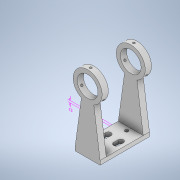
# Autodesk Inventor part: finderMainPartV05
Saved by Autodesk Inventor 2021 (Build 250183000, 183)
## iProperties
Created: 2020-06-05
Part Number: finderMainPartV05
Material: Generic
Document SubType Name: Modeling
Designer: robst
Density: 1 g/cm^3
Appearance: Default
Author: robst
Autodesk Inventor part; units mm, degrees
ref_plane "YZ Plane" through (0, 0, 0) normal (1, 0, 0) x (0, 1, 0)
ref_plane "XY Plane" through (0, 0, 0) normal (0, 0, 1) x (1, 0, 0)
sketch "Sketch1" plane through (0, 0, 0) normal (0, 0, 1) x (1, 0, 0)
  arc A0 (19.05, 73.7803) -> (-19.05, 73.7803) centre (0, 0) ccw
  line L0 (0, 86.4803) -> (19.05, 86.4803)
  line L1 (19.05, 86.4803) -> (19.05, 73.7803)
  line L2 (0, 76.2) -> (0, 86.4803) construction
  line L3 (0, 86.4803) -> (-19.05, 86.4803)
  line L4 (-19.05, 86.4803) -> (-19.05, 73.7803)
  dimension "d0" = 152.4
  dimension "d1" = 19.05
  dimension "d2" = 12.7
  constraints: 10 end point, 3 point on circle, 2 symmetric about line, 1 centre point, 1 coincident, 1 horizontal, 1 perpendicular, 1 vertical
  measures "d0" diameter of A0
  measures "d1" distance of L0.start L0.end
  measures "d2" distance of L0.end L1.end
extrude "Extrusion1" add sketch "Sketch1" along normal mid plane 75.6666
sketch "Sketch2" plane through (-19.05, 86.4803, 37.8333) normal (0, 1, 0) x (1, 0, 0)
  line L0 (0, 75.6666) -> (0, 0) construction
  line L1 (0, 37.8333) -> (38.1, 37.8333) construction
  line L2 (38.1, 75.6666) -> (38.1, 0) construction
  line L3 (0, 75.6666) -> (38.1, 75.6666) construction
  line L4 (19.05, 75.6666) -> (19.05, 0) construction
  line L5 (38.1, 0) -> (0, 0) construction
  line L6 (28.575, 34.3408) -> (28.575, 41.3258) construction
  line L7 (24.4475, 34.3408) -> (24.4475, 41.3258)
  line L8 (32.7025, 41.3258) -> (32.7025, 34.3408)
  arc A0 (24.4475, 34.3408) -> (32.7025, 34.3408) centre (28.575, 34.3408) ccw
  arc A1 (32.7025, 41.3258) -> (24.4475, 41.3258) centre (28.575, 41.3258) ccw
  line L9 (13.6525, 34.3408) -> (13.6525, 41.3258)
  line L10 (5.3975, 41.3258) -> (5.3975, 34.3408)
  arc A2 (5.3975, 34.3408) -> (13.6525, 34.3408) centre (9.525, 34.3408) ccw
  arc A3 (13.6525, 41.3258) -> (5.3975, 41.3258) centre (9.525, 41.3258) ccw
  point P0 (19.05, 37.8333)
  point P1 (28.575, 37.8333)
  dimension "d5" = 9.525
  dimension "d6" = 8.255
  dimension "d7" = 15.24
  dimension "d8" = 19.05
  dimension "d170" = 8.255
  constraints: 16 end point, 8 point on circle, 6 symmetric about line, 5 midpoint, 4 centre point, 4 tangent, 1 parallel, 1 perpendicular, 1 point on line, 2 other
  measures "d5" distance of point (28.575, 37.833) point (19.05, 37.833)
  measures "d6" distance between parallel lines of L8 L7
  measures "d8" distance of L6.end A3.centre
  measures "d170" distance between parallel lines of L9 L10
extrude "Extrusion2" cut sketch "Sketch2" against normal through all
ref_plane "Work Plane1" through (19.05, 73.7803, 37.8333) normal (0, 1, 0) x (-1, 0, 0)
sketch "Sketch5" plane through (0, 0, 37.8333) normal (0, 0, 1) x (1, 0, 0)
  circle A0 centre (0, 175.3803) radius 15.875
  arc A1 (9.525, 155.2999) -> (-9.525, 155.2999) centre (0, 175.3803) ccw
  arc A2 (19.05, 73.7803) -> (-19.05, 73.7803) centre (0, 0) ccw construction
  line L0 (-19.05, 73.7803) -> (19.05, 73.7803) construction
  line L1 (19.05, 86.4803) -> (9.525, 155.2999)
  line L2 (19.05, 86.4803) -> (-19.05, 86.4803) construction
  line L3 (0, 86.4803) -> (0, 175.3803) construction
  line L4 (-19.05, 86.4803) -> (-9.525, 155.2999)
  line L5 (-19.05, 86.4803) -> (19.05, 86.4803)
  dimension "d15" = 31.75
  dimension "d16" = 6.35
  dimension "d17" = 101.6
  dimension "d18" = 9.525
  constraints: 10 end point, 2 centre point, 2 horizontal, 2 point on circle, 1 coincident, 1 midpoint, 1 perpendicular, 1 symmetric about line
  measures "d15" diameter of A0
  measures "d16" radial gap between concentric circles of A1 A0
  measures "d17" distance from line of A0.centre L0
  measures "d18" distance from line of L1.end L3
extrude "Extrusion4" add sketch "Sketch5" against normal blind 9.525
ref_plane "Work Plane2" through (0, 197.6053, 37.8333) normal (0, 1, 0) x (-1, 0, 0)
sketch "Sketch6" plane through (0, 197.6053, 37.8333) normal (0, 1, 0) x (-1, 0, 0)
  line L0 (-22.225, -9.525) -> (22.225, -9.525) projected
  circle A0 centre (0, -4.7625) radius 1.7272
  point P0 (0, -37.8333)
  point P1 (9.525, -9.525)
  point P2 (-9.525, -9.525)
  dimension "d21" = 4.7625
  dimension "d22" = 3.4544
  constraints: 1 centre point
  measures "d21" distance from line of A0.centre L0
  measures "d22" diameter of A0
extrude "Extrusion5" cut sketch "Sketch6" against normal up to surface round surface about axis through (0, 175.3803, 37.8333) along (0, 0, -1) radius 15.875 far side no
pattern_circular "Circular Pattern1" count 3 over 360 about axis through (0, 175.3803, 37.8333) along (0, 0, -1) of "Extrusion5"
mirror "Mirror1" about plane through (0, 0, 0) normal (0, 0, 1) of "Extrusion4", "Extrusion5", "Circular Pattern1"
sketch "Sketch20" plane through (19.05, 73.7803, 37.8333) normal (1, 0, 0) x (0, 0, -1)
  line L0 (0, 12.7) -> (0, 0) projected
  line L1 (75.6666, 12.7) -> (75.6666, 0) projected
  line L2 (0, 0) -> (75.6666, 0)
  line L3 (75.6666, 0) -> (75.6666, 6.35)
  line L4 (75.6666, 6.35) -> (0, 6.35)
  line L5 (0, 6.35) -> (0, 0)
  point P0 (37.8333, -73.7803)
  point P1 (0, 6.35)
  constraints: 8 end point, 2 parallel, 1 horizontal, 1 midpoint, 1 perpendicular
extrude "Extrusion7" cut sketch "Sketch20" against normal through all
sketch "Sketch22" plane through (-19.05, 86.4803, 28.3083) normal (0, 1, 0) x (1, 0, 0)
  line L0 (41.275, 0) -> (-3.175, 0) projected
  line L1 (41.275, 56.6166) -> (-3.175, 56.6166) projected
  line L2 (-3.175, 66.1416) -> (41.275, 66.1416) projected
  point P0 (19.05, 28.3083)
  point P1 (19.05, 6.35)
  point P2 (19.05, 50.2666)
  point P3 (9.525, 0)
  point P4 (28.575, 0)
  point P5 (9.525, 56.6166)
  point P6 (28.575, 56.6166)
  point P7 (28.575, 66.1416)
  point P8 (9.525, 66.1416)
  dimension "d173" = 6.35
  dimension "d174" = 6.35
  dimension "d183" = 15.875
  measures "d173" distance from line of point (19.05, 6.35) L0
  measures "d174" distance from line of point (19.05, 50.267) L1
  measures "d183" distance from line of point (19.05, 50.267) L2
hole "Hole1" at (0, 86.4803, 21.9583) at (0, 86.4803, -21.9583) direction (0, -1, 0) diameter 5.1054 end through all clearance for "Socket Head Cap Screw" size "#10" standard "Ansi Unified Screw Threads"
equation "\"d51\" = 0.125 * Sketch8_Pitch"
equation "\"Sketch8_Pitch\" = 0.79375"
equation "\"d53\" = 60deg"
equation "\"d72\" = 0.125 * Sketch10_Pitch"
equation "\"Sketch10_Pitch\" = 0.79375"
equation "\"d74\" = 60deg"
equation "\"d93\" = 0.125 * Sketch12_Pitch"
equation "\"Sketch12_Pitch\" = 0.79375"
equation "\"d95\" = 60deg"
equation "\"d114\" = 0.125 * Sketch14_Pitch"
equation "\"Sketch14_Pitch\" = 0.79375"
equation "\"d116\" = 60deg"
equation "\"d135\" = 0.125 * Sketch16_Pitch"
equation "\"Sketch16_Pitch\" = 0.79375"
equation "\"d137\" = 60deg"
equation "\"d156\" = 0.125 * Sketch18_Pitch"
equation "\"Sketch18_Pitch\" = 0.79375"
equation "\"d158\" = 60deg"
body "Solid1"
